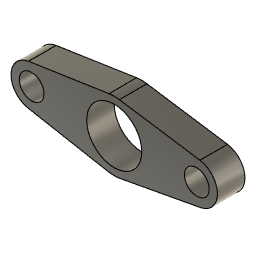
Part 10 (Autodesk Fusion 360 design; units mm, degrees)
Autodesk Fusion 360 part; units mm, degrees
sketch "Sketch2" plane through (0, 0, 0) normal (0, 1, 0) x (1, 0, 0)
  line L0 (-75, -1.0078) -> (75, -1.0078) construction
  line L1 (3.752, -24.7168) -> (62.2428, -15.8379)
  line L2 (-3.752, -24.7168) -> (-62.2428, -15.8379)
  line L3 (-4.5801, 24.5769) -> (-62.7396, 13.7383)
  line L4 (4.5801, 24.5769) -> (62.7396, 13.7383)
  arc A0 (62.2428, -15.8379) -> (62.7396, 13.7383) centre (59.9915, -1.0078) ccw
  arc A1 (-62.7396, 13.7383) -> (-62.2428, -15.8379) centre (-59.9915, -1.0078) ccw
  arc A2 (-3.752, -24.7168) -> (3.752, -24.7168) centre (0, 0) ccw
  arc A3 (4.5801, 24.5769) -> (-4.5801, 24.5769) centre (0, 0) ccw
  circle A4 centre (0, 0) radius 20
  circle A5 centre (59.9915, -1.0078) radius 9
  circle A6 centre (-59.9915, -1.0078) radius 9
  dimension "d8" = 50
  dimension "d9" = 30
  dimension "d10" = 30
  dimension "d11" = 60
  dimension "d12" = 60
  dimension "d13" = 40
  dimension "d14" = 18
  dimension "d15" = 18
  constraint horizontal L0
  constraint coincident A2.centre A3.centre
  constraint coincident L0 A0.centre
  constraint coincident L0 A1.centre
  constraint tangent L1 A0
  constraint tangent L1 A2
  constraint tangent L4 A0
  constraint tangent L4 A2
  constraint tangent L3 A1
  constraint tangent L3 A2
  constraint tangent L2 A2
  constraint tangent L2 A1
  constraint coincident L4.start A2
  constraint concentric A2 A3
  constraint concentric A3 A4
  constraint concentric A0 A5
  constraint concentric A1 A6
  measures "d8" diameter of A2
  measures "d9" diameter of A0
  measures "d10" diameter of A1
  measures "d11" distance of A2.centre A1.centre
  measures "d12" distance of A2.centre A0.centre
  measures "d13" diameter of A4
  measures "d14" diameter of A5
  measures "d15" diameter of A6
extrude "Extrude1" add sketch "Sketch2" along normal blind 20
